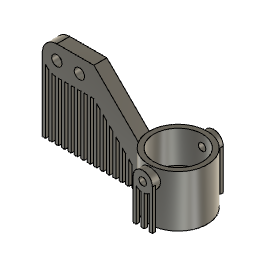
WheelArm12by4mm v7 (Autodesk Fusion 360 design; units mm, degrees)
Autodesk Fusion 360 part; units mm, degrees
note: some values were not read from the file. Set by a fixed rule: which sketch regions a step uses.
sketch "Sketch1" plane through (0, 0, 0) normal (0, 0, 1) x (1, 0, 0)
  circle A0 centre (0, 0) radius 6.25
  circle A1 centre (0, 0) radius 5
  circle A2 centre (0, 0) radius 7.5
  circle A3 centre (0, 0) radius 9
  dimension "d1" = 12.5
  dimension "d2" = 10
  dimension "d3" = 15
  dimension "d10" = 18
  constraint coincident A0.centre A1.centre
  constraint concentric A0 A2
  constraint concentric A1 A3
  measures "d1" diameter of A0
  measures "d2" diameter of A1
  measures "d3" diameter of A2
  measures "d10" diameter of A3
extrude "Extrude1" add sketch "Sketch1" along normal blind 2 contours A0
extrude "Extrude2" add sketch "Sketch1" along normal blind 6 contours A2
extrude "Extrude4" add sketch "Sketch1" along normal blind 16 contours A3
sketch "Sketch2" plane through (0, 0, 0) normal (0, 1, 0) x (1, 0, 0)
  circle A0 centre (0, -12.5) radius 1.15
  circle A1 centre (0, -12.5) radius 3
  dimension "d14" = 2.3
  dimension "d15" = 6
  measures "d14" diameter of A0
  measures "d15" diameter of A1
extrude "Extrude5" add sketch "Sketch2" along normal blind 3 from surface at 8
extrude "Extrude6" add sketch "Sketch2" along normal blind 3 from surface at -11
extrude "Extrude7" cut sketch "Sketch2" along normal blind 4 from surface at 7 contours A0
extrude "Extrude8" cut sketch "Sketch2" along normal blind 4 from surface at -11 contours A0
sketch "Sketch3" plane through (0, 0, 0) normal (0, 1, 0) x (1, 0, 0)
  line L0 (-8, -13) -> (-10, -13)
  line L1 (-10, -13) -> (-10, -4)
  line L2 (-10, -4) -> (-8, -4)
  line L3 (-8, -4) -> (-8, -13)
  line L4 (-10, -8.5) -> (-24.1421, -22.6421)
  line L5 (-10, -8.5) -> (10, -8.5) construction
  line L6 (-10, -4) -> (-24.1421, -18.1421)
  line L7 (-10, -4) -> (10, -4) construction
  line L8 (-10, -13) -> (-24.1421, -27.1421)
  line L9 (-10, -13) -> (10, -13) construction
  line L10 (-24.1421, -18.1421) -> (-24.1421, -27.1421)
  line L11 (-24.1421, -27.1421) -> (-40.1421, -27.1421)
  line L12 (-40.1421, -27.1421) -> (-40.1421, -18.1421)
  line L13 (-40.1421, -18.1421) -> (-24.1421, -18.1421)
  line L14 (-24.1421, -18.1421) -> (-24.1421, -27.1421)
  line L15 (-24.1421, -22.6421) -> (-28.6421, -22.6421)
  circle A0 centre (-28.6421, -22.6421) radius 1.6
  line L16 (-28.6421, -22.6421) -> (-35.6421, -22.6421)
  circle A1 centre (-28.6421, -22.6421) radius 4.5
  circle A2 centre (-35.6421, -22.6421) radius 1.6
  circle A3 centre (-35.6421, -22.6421) radius 4.5
  dimension "d28" = 2
  dimension "d29" = 9
  dimension "d30" = 135
  dimension "d31" = 20
  dimension "d32" = 135
  dimension "d33" = 20
  dimension "d34" = 135
  dimension "d35" = 20
  dimension "d36" = 16
  dimension "d37" = 9
  dimension "d38" = 4.5
  dimension "d39" = 3.2
  dimension "d40" = 7
  dimension "d42" = 9
  dimension "d43" = 3.2
  dimension "d44" = 9
  constraint horizontal L0
  constraint vertical L1
  constraint horizontal L2
  constraint vertical L3
  constraint horizontal L5
  constraint midpoint L1 L4.start
  constraint horizontal L7
  constraint horizontal L9
  constraint horizontal L11
  constraint vertical L12
  constraint horizontal L13
  constraint vertical L14
  constraint coincident L15.end A0.centre
  constraint parallel L15 L16
  constraint coincident L16.end A2.centre
  constraint concentric A2 A3
  measures "d28" distance of L0.start L0.end
  measures "d29" distance of L0.start L2.end
  measures "d30" angle of L4 L5
  measures "d31" distance of L4.start L4.end
  measures "d32" angle of L6 L7
  measures "d33" distance of L1.end L6.end
  measures "d34" angle of L8 L9
  measures "d35" distance of L0.end L8.end
  measures "d36" distance of L8.end L11.end
  measures "d37" distance of L8.end L6.end
  measures "d38" distance of L4.end L15.end
  measures "d39" diameter of A0
  measures "d40" distance of L15.end L16.end
  measures "d42" diameter of A1
  measures "d43" diameter of A2
  measures "d44" diameter of A3
extrude "Extrude9" add sketch "Sketch3" along normal mid plane 4 contours L0 L1 L2 L3 | L1 L4 L8 L10 L14 | L1 L4 L6 L10 L14 | L10 L11 L14 A1 | L10 L13 L14 A1 | L15 A0 L16 A1 A3 | L15 A0 L16 A1 A3 | L11 A1 A3 | L13 A1 A3 | A1 A3 | L16 A1 A3 | L16 A1 A3
sketch "Sketch4" plane through (0, 0, 0) normal (0, 0, 1) x (1, 0, 0)
  line L0 (-3, 11) -> (-2, 11)
  line L1 (-2, 11) -> (-2, 10)
  line L2 (-2, 10) -> (-3, 10)
  line L3 (-3, 10) -> (-3, 11)
  line L4 (-0.5, 10) -> (-0.5, 11)
  line L5 (-0.5, 11) -> (0.5, 11)
  line L6 (0.5, 10) -> (-0.5, 10)
  line L7 (0.5, 11) -> (0.5, 10)
  line L8 (2, 10) -> (2, 11)
  line L9 (2, 11) -> (3, 11)
  line L10 (3, 10) -> (2, 10)
  line L11 (3, 11) -> (3, 10)
  line L12 (-3, -11) -> (-2, -11)
  line L13 (-2, -11) -> (-2, -10)
  line L14 (-2, -10) -> (-3, -10)
  line L15 (-3, -10) -> (-3, -11)
  line L16 (-0.5, -10) -> (-0.5, -11)
  line L17 (-0.5, -11) -> (0.5, -11)
  line L18 (0.5, -10) -> (-0.5, -10)
  line L19 (0.5, -11) -> (0.5, -10)
  line L20 (2, -10) -> (2, -11)
  line L21 (2, -11) -> (3, -11)
  line L22 (3, -10) -> (2, -10)
  line L23 (3, -11) -> (3, -10)
  line L24 (-40.1425, -2) -> (-39.1425, -2)
  line L25 (-39.1425, -2) -> (-39.1425, -1)
  line L26 (-39.1425, -1) -> (-40.1425, -1)
  line L27 (-40.1425, -1) -> (-40.1425, -2)
  line L28 (-38.1558, -2) -> (-37.1558, -2)
  line L29 (-37.1558, -2) -> (-37.1558, -1)
  line L30 (-38.1558, -1) -> (-38.1558, -2)
  line L31 (-37.1558, -1) -> (-38.1558, -1)
  line L32 (-36.1692, -2) -> (-35.1692, -2)
  line L33 (-35.1692, -2) -> (-35.1692, -1)
  line L34 (-36.1692, -1) -> (-36.1692, -2)
  line L35 (-35.1692, -1) -> (-36.1692, -1)
  line L36 (-34.1825, -2) -> (-33.1825, -2)
  line L37 (-33.1825, -2) -> (-33.1825, -1)
  line L38 (-34.1825, -1) -> (-34.1825, -2)
  line L39 (-33.1825, -1) -> (-34.1825, -1)
  line L40 (-32.1958, -2) -> (-31.1958, -2)
  line L41 (-31.1958, -2) -> (-31.1958, -1)
  line L42 (-32.1958, -1) -> (-32.1958, -2)
  line L43 (-31.1958, -1) -> (-32.1958, -1)
  line L44 (-30.2092, -2) -> (-29.2092, -2)
  line L45 (-29.2092, -2) -> (-29.2092, -1)
  line L46 (-30.2092, -1) -> (-30.2092, -2)
  line L47 (-29.2092, -1) -> (-30.2092, -1)
  line L48 (-28.2225, -2) -> (-27.2225, -2)
  line L49 (-27.2225, -2) -> (-27.2225, -1)
  line L50 (-28.2225, -1) -> (-28.2225, -2)
  line L51 (-27.2225, -1) -> (-28.2225, -1)
  line L52 (-26.2358, -2) -> (-25.2358, -2)
  line L53 (-25.2358, -2) -> (-25.2358, -1)
  line L54 (-26.2358, -1) -> (-26.2358, -2)
  line L55 (-25.2358, -1) -> (-26.2358, -1)
  line L56 (-24.2492, -2) -> (-23.2492, -2)
  line L57 (-23.2492, -2) -> (-23.2492, -1)
  line L58 (-24.2492, -1) -> (-24.2492, -2)
  line L59 (-23.2492, -1) -> (-24.2492, -1)
  line L60 (-22.2625, -2) -> (-21.2625, -2)
  line L61 (-21.2625, -2) -> (-21.2625, -1)
  line L62 (-22.2625, -1) -> (-22.2625, -2)
  line L63 (-21.2625, -1) -> (-22.2625, -1)
  line L64 (-20.2758, -2) -> (-19.2758, -2)
  line L65 (-19.2758, -2) -> (-19.2758, -1)
  line L66 (-20.2758, -1) -> (-20.2758, -2)
  line L67 (-19.2758, -1) -> (-20.2758, -1)
  line L68 (-18.2892, -2) -> (-17.2892, -2)
  line L69 (-17.2892, -2) -> (-17.2892, -1)
  line L70 (-18.2892, -1) -> (-18.2892, -2)
  line L71 (-17.2892, -1) -> (-18.2892, -1)
  line L72 (-16.3025, -2) -> (-15.3025, -2)
  line L73 (-15.3025, -2) -> (-15.3025, -1)
  line L74 (-16.3025, -1) -> (-16.3025, -2)
  line L75 (-15.3025, -1) -> (-16.3025, -1)
  line L76 (-14.3158, -2) -> (-13.3158, -2)
  line L77 (-13.3158, -2) -> (-13.3158, -1)
  line L78 (-14.3158, -1) -> (-14.3158, -2)
  line L79 (-13.3158, -1) -> (-14.3158, -1)
  line L80 (-12.3292, -2) -> (-11.3292, -2)
  line L81 (-11.3292, -2) -> (-11.3292, -1)
  line L82 (-12.3292, -1) -> (-12.3292, -2)
  line L83 (-11.3292, -1) -> (-12.3292, -1)
  line L84 (-10.3425, -2) -> (-9.3425, -2)
  line L85 (-9.3425, -2) -> (-9.3425, -1)
  line L86 (-10.3425, -1) -> (-10.3425, -2)
  line L87 (-9.3425, -1) -> (-10.3425, -1)
  line L88 (-40.1425, -0.5) -> (-39.1425, -0.5)
  line L89 (-39.1425, -0.5) -> (-39.1425, 0.5)
  line L90 (-40.1425, 0.5) -> (-40.1425, -0.5)
  line L91 (-39.1425, 0.5) -> (-40.1425, 0.5)
  line L92 (-38.1558, -0.5) -> (-37.1558, -0.5)
  line L93 (-37.1558, -0.5) -> (-37.1558, 0.5)
  line L94 (-38.1558, 0.5) -> (-38.1558, -0.5)
  line L95 (-37.1558, 0.5) -> (-38.1558, 0.5)
  line L96 (-36.1692, -0.5) -> (-35.1692, -0.5)
  line L97 (-35.1692, -0.5) -> (-35.1692, 0.5)
  line L98 (-36.1692, 0.5) -> (-36.1692, -0.5)
  line L99 (-35.1692, 0.5) -> (-36.1692, 0.5)
  line L100 (-34.1825, -0.5) -> (-33.1825, -0.5)
  line L101 (-33.1825, -0.5) -> (-33.1825, 0.5)
  line L102 (-34.1825, 0.5) -> (-34.1825, -0.5)
  line L103 (-33.1825, 0.5) -> (-34.1825, 0.5)
  line L104 (-32.1958, -0.5) -> (-31.1958, -0.5)
  line L105 (-31.1958, -0.5) -> (-31.1958, 0.5)
  line L106 (-32.1958, 0.5) -> (-32.1958, -0.5)
  line L107 (-31.1958, 0.5) -> (-32.1958, 0.5)
  line L108 (-30.2092, -0.5) -> (-29.2092, -0.5)
  line L109 (-29.2092, -0.5) -> (-29.2092, 0.5)
  line L110 (-30.2092, 0.5) -> (-30.2092, -0.5)
  line L111 (-29.2092, 0.5) -> (-30.2092, 0.5)
  line L112 (-28.2225, -0.5) -> (-27.2225, -0.5)
  line L113 (-27.2225, -0.5) -> (-27.2225, 0.5)
  line L114 (-28.2225, 0.5) -> (-28.2225, -0.5)
  line L115 (-27.2225, 0.5) -> (-28.2225, 0.5)
  line L116 (-26.2358, -0.5) -> (-25.2358, -0.5)
  line L117 (-25.2358, -0.5) -> (-25.2358, 0.5)
  line L118 (-26.2358, 0.5) -> (-26.2358, -0.5)
  line L119 (-25.2358, 0.5) -> (-26.2358, 0.5)
  line L120 (-24.2492, -0.5) -> (-23.2492, -0.5)
  line L121 (-23.2492, -0.5) -> (-23.2492, 0.5)
  line L122 (-24.2492, 0.5) -> (-24.2492, -0.5)
  line L123 (-23.2492, 0.5) -> (-24.2492, 0.5)
  line L124 (-22.2625, -0.5) -> (-21.2625, -0.5)
  line L125 (-21.2625, -0.5) -> (-21.2625, 0.5)
  line L126 (-22.2625, 0.5) -> (-22.2625, -0.5)
  line L127 (-21.2625, 0.5) -> (-22.2625, 0.5)
  line L128 (-20.2758, -0.5) -> (-19.2758, -0.5)
  line L129 (-19.2758, -0.5) -> (-19.2758, 0.5)
  line L130 (-20.2758, 0.5) -> (-20.2758, -0.5)
  line L131 (-19.2758, 0.5) -> (-20.2758, 0.5)
  line L132 (-18.2892, -0.5) -> (-17.2892, -0.5)
  line L133 (-17.2892, -0.5) -> (-17.2892, 0.5)
  line L134 (-18.2892, 0.5) -> (-18.2892, -0.5)
  line L135 (-17.2892, 0.5) -> (-18.2892, 0.5)
  line L136 (-16.3025, -0.5) -> (-15.3025, -0.5)
  line L137 (-15.3025, -0.5) -> (-15.3025, 0.5)
  line L138 (-16.3025, 0.5) -> (-16.3025, -0.5)
  line L139 (-15.3025, 0.5) -> (-16.3025, 0.5)
  line L140 (-14.3158, -0.5) -> (-13.3158, -0.5)
  line L141 (-13.3158, -0.5) -> (-13.3158, 0.5)
  line L142 (-14.3158, 0.5) -> (-14.3158, -0.5)
  line L143 (-13.3158, 0.5) -> (-14.3158, 0.5)
  line L144 (-12.3292, -0.5) -> (-11.3292, -0.5)
  line L145 (-11.3292, -0.5) -> (-11.3292, 0.5)
  line L146 (-12.3292, 0.5) -> (-12.3292, -0.5)
  line L147 (-11.3292, 0.5) -> (-12.3292, 0.5)
  line L148 (-10.3425, -0.5) -> (-9.3425, -0.5)
  line L149 (-9.3425, -0.5) -> (-9.3425, 0.5)
  line L150 (-10.3425, 0.5) -> (-10.3425, -0.5)
  line L151 (-9.3425, 0.5) -> (-10.3425, 0.5)
  line L152 (-40.1425, 1) -> (-39.1425, 1)
  line L153 (-39.1425, 1) -> (-39.1425, 2)
  line L154 (-40.1425, 2) -> (-40.1425, 1)
  line L155 (-39.1425, 2) -> (-40.1425, 2)
  line L156 (-38.1558, 1) -> (-37.1558, 1)
  line L157 (-37.1558, 1) -> (-37.1558, 2)
  line L158 (-38.1558, 2) -> (-38.1558, 1)
  line L159 (-37.1558, 2) -> (-38.1558, 2)
  line L160 (-36.1692, 1) -> (-35.1692, 1)
  line L161 (-35.1692, 1) -> (-35.1692, 2)
  line L162 (-36.1692, 2) -> (-36.1692, 1)
  line L163 (-35.1692, 2) -> (-36.1692, 2)
  line L164 (-34.1825, 1) -> (-33.1825, 1)
  line L165 (-33.1825, 1) -> (-33.1825, 2)
  line L166 (-34.1825, 2) -> (-34.1825, 1)
  line L167 (-33.1825, 2) -> (-34.1825, 2)
  line L168 (-32.1958, 1) -> (-31.1958, 1)
  line L169 (-31.1958, 1) -> (-31.1958, 2)
  line L170 (-32.1958, 2) -> (-32.1958, 1)
  line L171 (-31.1958, 2) -> (-32.1958, 2)
  line L172 (-30.2092, 1) -> (-29.2092, 1)
  line L173 (-29.2092, 1) -> (-29.2092, 2)
  line L174 (-30.2092, 2) -> (-30.2092, 1)
  line L175 (-29.2092, 2) -> (-30.2092, 2)
  line L176 (-28.2225, 1) -> (-27.2225, 1)
  line L177 (-27.2225, 1) -> (-27.2225, 2)
  line L178 (-28.2225, 2) -> (-28.2225, 1)
  line L179 (-27.2225, 2) -> (-28.2225, 2)
  line L180 (-26.2358, 1) -> (-25.2358, 1)
  line L181 (-25.2358, 1) -> (-25.2358, 2)
  line L182 (-26.2358, 2) -> (-26.2358, 1)
  line L183 (-25.2358, 2) -> (-26.2358, 2)
  line L184 (-24.2492, 1) -> (-23.2492, 1)
  line L185 (-23.2492, 1) -> (-23.2492, 2)
  line L186 (-24.2492, 2) -> (-24.2492, 1)
  line L187 (-23.2492, 2) -> (-24.2492, 2)
  line L188 (-22.2625, 1) -> (-21.2625, 1)
  line L189 (-21.2625, 1) -> (-21.2625, 2)
  line L190 (-22.2625, 2) -> (-22.2625, 1)
  line L191 (-21.2625, 2) -> (-22.2625, 2)
  line L192 (-20.2758, 1) -> (-19.2758, 1)
  line L193 (-19.2758, 1) -> (-19.2758, 2)
  line L194 (-20.2758, 2) -> (-20.2758, 1)
  line L195 (-19.2758, 2) -> (-20.2758, 2)
  line L196 (-18.2892, 1) -> (-17.2892, 1)
  line L197 (-17.2892, 1) -> (-17.2892, 2)
  line L198 (-18.2892, 2) -> (-18.2892, 1)
  line L199 (-17.2892, 2) -> (-18.2892, 2)
  line L200 (-16.3025, 1) -> (-15.3025, 1)
  line L201 (-15.3025, 1) -> (-15.3025, 2)
  line L202 (-16.3025, 2) -> (-16.3025, 1)
  line L203 (-15.3025, 2) -> (-16.3025, 2)
  line L204 (-14.3158, 1) -> (-13.3158, 1)
  line L205 (-13.3158, 1) -> (-13.3158, 2)
  line L206 (-14.3158, 2) -> (-14.3158, 1)
  line L207 (-13.3158, 2) -> (-14.3158, 2)
  line L208 (-12.3292, 1) -> (-11.3292, 1)
  line L209 (-11.3292, 1) -> (-11.3292, 2)
  line L210 (-12.3292, 2) -> (-12.3292, 1)
  line L211 (-11.3292, 2) -> (-12.3292, 2)
  line L212 (-10.3425, 1) -> (-9.3425, 1)
  line L213 (-9.3425, 1) -> (-9.3425, 2)
  line L214 (-10.3425, 2) -> (-10.3425, 1)
  line L215 (-9.3425, 2) -> (-10.3425, 2)
  dimension "d49" = 5
  dimension "d50" = 0
  dimension "d51" = 1
  dimension "d52" = 1
  dimension "d55" = 5
  dimension "d56" = 0
  dimension "d57" = 1
  dimension "d58" = 1
  dimension "d61" = 29.8
  dimension "d62" = 3
  constraint horizontal L0
  constraint vertical L1
  constraint horizontal L2
  constraint vertical L3
  constraint horizontal L12
  constraint vertical L13
  constraint horizontal L14
  constraint vertical L15
  constraint horizontal L24
  constraint vertical L25
  constraint horizontal L26
  constraint vertical L27
  measures "d51" distance of L12.start L12.end
  measures "d52" distance of L12.start L14.end
  measures "d57" distance of L24.start L24.end
  measures "d58" distance of L24.start L26.end
extrude "Extrude10" add sketch "Sketch4" along normal blind 12.5 contours L12 L13 L14 L15 | L20 L21 L22 L23
extrude "Extrude11" add sketch "Sketch4" along normal blind 12.5 contours L0 L1 L2 L3 | L8 L9 L10 L11
extrude "Extrude12" add sketch "Sketch4" along normal blind 10 contours L4 L5 L6 L7
extrude "Extrude13" add sketch "Sketch4" along normal blind 10 contours L16 L17 L18 L19
extrude "Extrude14" add sketch "Sketch4" along normal blind 23 contours L24 L25 L26 L27 | L88 L89 L90 L91 | L152 L153 L154 L155
extrude "Extrude15" add sketch "Sketch4" along normal blind 20 contours L28 L29 L30 L31 | L32 L33 L34 L35 | L36 L37 L38 L39 | L40 L41 L42 L43 | L44 L45 L46 L47 | L48 L49 L50 L51 | L52 L53 L54 L55 | L56 L57 L58 L59 | L60 L61 L62 L63 | L64 L65 L66 L67 | L68 L69 L70 L71 | L92 L93 L94 L95 | L96 L97 L98 L99 | L100 L101 L102 L103 | L104 L105 L106 L107 | L108 L109 L110 L111 | L112 L113 L114 L115 | L116 L117 L118 L119 | L120 L121 L122 L123 | L124 L125 L126 L127 | L128 L129 L130 L131 | L132 L133 L134 L135 | L156 L157 L158 L159 | L160 L161 L162 L163 | L164 L165 L166 L167 | L168 L169 L170 L171 | L172 L173 L174 L175 | L176 L177 L178 L179 | L180 L181 L182 L183 | L184 L185 L186 L187 | L188 L189 L190 L191 | L192 L193 L194 L195 | L196 L197 L198 L199
extrude "Extrude16" add sketch "Sketch4" along normal blind 11 contours L72 L73 L74 L75 | L76 L77 L78 L79 | L80 L81 L82 L83 | L84 L85 L86 L87 | L136 L137 L138 L139 | L140 L141 L142 L143 | L144 L145 L146 L147 | L148 L149 L150 L151 | L200 L201 L202 L203 | L204 L205 L206 L207 | L208 L209 L210 L211 | L212 L213 L214 L215
equation "d11 = 6 mm + 7 mm + 3 mm"
equation "d19 = -8 mm - 3 mm"
equation "d25 = -8 mm - 3 mm"
equation "d63 = 9.50 mm + 3 mm"
equation "d65 = 9.5 mm + 3 mm"
equation "d67 = 7 mm + 3 mm"
equation "d69 = 7 mm + 3 mm"
named bodies: "BratRefacut"
